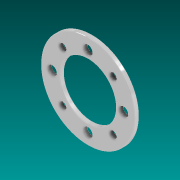
# Autodesk Inventor part: afstandsplaatje
Saved by Autodesk Inventor 2020.2 (Build 242310000, 310)
## iProperties
Created: 2020-05-15
Part Number: afstandsplaatje
Material: Aluminum 6061
Document SubType Name: Modeling
Designer: Svend
Density: 2.7 g/cm^3
Appearance: Aluminum - Polished
Author: Svend
Autodesk Inventor part; units mm, degrees
ref_plane "YZ Plane" through (0, 0, 0) normal (1, 0, 0) x (0, 1, 0)
ref_plane "XZ Plane" through (0, 0, 0) normal (0, 1, 0) x (-1, 0, 0)
ref_plane "XY Plane" through (0, 0, 0) normal (0, 0, 1) x (1, 0, 0)
sketch "Sketch1" plane through (0, 0, 0) normal (0, 0, 1) x (1, 0, 0)
  circle A0 centre (0, 0) radius 21
  circle A1 centre (16, 0) radius 2
  circle A2 centre (0, 16) radius 2
  circle A3 centre (-16, 0) radius 2
  circle A4 centre (0, -16) radius 2
  line L0 (-14.8492, -14.8492) -> (14.8492, 14.8492)
  line L1 (0, -21) -> (0, 21)
  circle A5 centre (11.3137, 11.3137) radius 1.5
  circle A6 centre (-11.3137, 11.3137) radius 1.5
  circle A7 centre (-11.3137, -11.3137) radius 1.5
  circle A8 centre (11.3137, -11.3137) radius 1.5
  circle A9 centre (0, 0) radius 12.6
  dimension "d0" = 42
  dimension "d1" = 4
  dimension "d5" = 16
  dimension "d8" = 360
  dimension "d10" = 45
  dimension "d11" = 3
  dimension "d12" = 16
  dimension "d15" = 360
  dimension "d19" = 25.2
  constraints: 10 centre point, 4 end point, 4 point on circle, 3 midpoint, 2 coincident, 1 horizontal alignment, 1 point on line, 1 vertical, 18 other
  measures "d0" diameter of A0
  measures "d1" diameter of A1
  measures "d5" distance of point (0, 0) A1.centre
  measures "d10" angle of L1 L0
  measures "d11" diameter of A5
  measures "d12" distance of point (0, 0) A5.centre
  measures "d19" diameter of A9
extrude "Extrusion1" add sketch "Sketch1" along normal blind 2 contours A0 L1 A4 A9 L0 A5 | L0 A5 A9 L1 A2 A0 | A0 L0 A7 A9 L1 A4 | L1 A2 A9 L0 A7 A0
chamfer "Chamfer1" distance 0.2 angle 45 20 edges at (-21, 0, 0) (-21, 0, 2) (-12.6, 0, 0) (-12.6, 0, 2) (-2, 16, 0) (-2, 16, 2) (-18, 0, 0) (-18, 0, 2) (-12.8137, 11.3137, 0) (-12.8137, 11.3137, 2) (-12.8137, -11.3137, 0) (-12.8137, -11.3137, 2) (9.8137, 11.3137, 0) (9.8137, 11.3137, 2) (14, 0, 0) (14, 0, 2) (9.8137, -11.3137, 0) (9.8137, -11.3137, 2) (-2, -16, 0) (-2, -16, 2)
body "Solid1"
